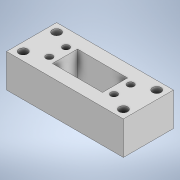
# Autodesk Inventor part: MotorHolder
Saved by Autodesk Inventor 2020.4 (Build 244396010, 396A)
## iProperties
Created: 2022-10-04
Part Number: MotorHolder
Material: Generic
Document SubType Name: Modeling
Designer: YUSTE
Density: 1 g/cm^3
Appearance: Default
Author: YUSTE
Autodesk Inventor part; units mm, degrees
ref_plane "YZ Plane" through (0, 0, 0) normal (1, 0, 0) x (0, 1, 0)
ref_plane "XZ Plane" through (0, 0, 0) normal (0, 1, 0) x (-1, 0, 0)
ref_plane "XY Plane" through (0, 0, 0) normal (0, 0, 1) x (1, 0, 0)
sketch "Sketch1" plane through (0, 0, 0) normal (0, 1, 0) x (-1, 0, 0)
  line L0 (0, 0) -> (0, 38.1)
  line L1 (0, 38.1) -> (88.9, 38.1)
  line L2 (88.9, 38.1) -> (88.9, 0)
  line L3 (88.9, 0) -> (0, 0)
  circle A0 centre (19.8437, 12.7) radius 2.54
  circle A1 centre (19.8437, 25.4) radius 2.54
  circle A2 centre (69.0563, 25.4) radius 2.54
  circle A3 centre (69.0563, 12.7) radius 2.54
  circle A4 centre (6.35, 31.75) radius 3.302
  circle A5 centre (6.35, 6.35) radius 3.302
  circle A6 centre (82.55, 31.75) radius 3.302
  circle A7 centre (82.55, 6.35) radius 3.302
  line L4 (63.5, 28.575) -> (63.5, 9.525)
  line L5 (63.5, 9.525) -> (25.4, 9.525)
  line L6 (25.4, 9.525) -> (25.4, 28.575)
  line L7 (25.4, 28.575) -> (63.5, 28.575)
  dimension "d0" = 38.1
  dimension "d1" = 88.9
  dimension "d2" = 5.08
  dimension "d3" = 5.08
  dimension "d4" = 5.08
  dimension "d5" = 5.08
  dimension "d6" = 12.7
  dimension "d7" = 12.7
  dimension "d8" = 12.7
  dimension "d9" = 12.7
  dimension "d10" = 49.2125
  dimension "d11" = 49.2125
  dimension "d12" = 19.8438
  dimension "d14" = 19.8438
  dimension "d15" = 6.604
  dimension "d16" = 6.604
  dimension "d17" = 6.604
  dimension "d18" = 6.604
  dimension "d19" = 25.4
  dimension "d20" = 6.35
  dimension "d21" = 6.35
  dimension "d22" = 6.35
  dimension "d23" = 6.35
  dimension "d24" = 6.35
  dimension "d25" = 25.4
  dimension "d26" = 6.35
  dimension "d27" = 19.05
  dimension "d28" = 38.1
  dimension "d29" = 9.525
  dimension "d30" = 25.4
  dimension "d33" = 6.35
  dimension "d34" = 76.2
  constraints: 16 end point, 8 centre point, 4 parallel, 2 perpendicular, 2 vertical
  measures "d0" distance of L0.start L0.end
  measures "d1" distance of L0.end L1.end
  measures "d2" diameter of A0
  measures "d3" diameter of A1
  measures "d4" diameter of A2
  measures "d5" diameter of A3
  measures "d6" distance of A0.centre A1.centre
  measures "d7" distance of A3.centre A2.centre
  measures "d8" distance from line of L1 A1.centre
  measures "d9" distance from line of L3 A3.centre
  measures "d10" distance of A1.centre A2.centre
  measures "d11" distance of A0.centre A3.centre
  measures "d12" distance from line of L0 A1.centre
  measures "d14" distance from line of L2 A3.centre
  measures "d15" diameter of A4
  measures "d16" diameter of A5
  measures "d17" diameter of A6
  measures "d18" diameter of A7
  measures "d19" distance of A4.centre A5.centre
  measures "d20" distance from line of L1 A4.centre
  measures "d21" distance from line of L0 A4.centre
  measures "d22" distance from line of L0 A5.centre
  measures "d23" distance from line of L2 A6.centre
  measures "d24" distance from line of L2 A7.centre
  measures "d25" distance of A7.centre A6.centre
  measures "d26" distance from line of L1 A6.centre
  measures "d27" distance of L4.start L4.end
  measures "d28" distance of L4.end L5.end
  measures "d29" distance between parallel lines of L1 L7
  measures "d30" distance between parallel lines of L0 L6
  measures "d33" distance from line of L3 A5.centre
  measures "d34" distance of A7.centre A5.centre
extrude "Extrusion1" add sketch "Sketch1" along normal blind 25.4
body "Solid1"
